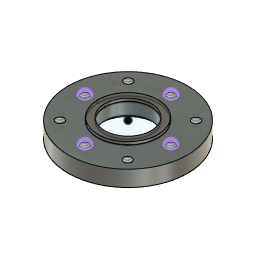
Driveshaft_adapter v1 (Autodesk Fusion 360 design; units mm, degrees)
Autodesk Fusion 360 part; units mm, degrees
note: some values were not read from the file. Set by a fixed rule: which sketch regions a step uses.
sketch "Big end" plane through (0, 0, 0) normal (0, 0, 1) x (1, 0, 0)
  circle A0 centre (0, 0) radius 75
  circle A1 centre (0, 0) radius 60.5 construction
  line L0 (-42.6, 42.9592) -> (42.6, 42.9592) construction
  line L1 (42.6, 42.9592) -> (42.6, -42.2408) construction
  line L2 (42.6, -42.2408) -> (-42.6, -42.2408) construction
  line L3 (-42.6, -42.2408) -> (-42.6, 42.9592) construction
  line L4 (42.6, 42.9592) -> (0, 0) construction
  line L5 (0, 0) -> (60.5, 0) construction
  circle A2 centre (-42.6, 42.9592) radius 6
  circle A3 centre (-42.9592, -42.6) radius 6
  circle A4 centre (42.6, -42.9592) radius 6
  circle A5 centre (42.9592, 42.6) radius 6
  circle A6 centre (0, 0) radius 54 construction
  circle A7 centre (54, 0) radius 6
  circle A8 centre (0, 54) radius 6
  circle A9 centre (-54, 0) radius 6
  circle A10 centre (0, -54) radius 6
  dimension "d1" = 150
  dimension "d2" = 121
  dimension "d4" = 85.2
  dimension "d5" = 85.2
  dimension "d6" = 12
  dimension "d8" = 360
  dimension "d15" = 108
  dimension "d16" = 12
  dimension "d18" = 360
  constraint coincident A0.centre A1.centre
  constraint concentric A0 A1
  constraint horizontal L0
  constraint vertical L1
  constraint horizontal L2
  constraint vertical L3
  constraint coincident A1 L0.start
  constraint coincident A1 L0.end
  constraint coincident A1 L5.end
  constraint perpendicular L1 L5
  constraint coincident L0.start L3.end
  constraint concentric A1 A6
  constraint coincident A6 A7.centre
  constraint coincident L5 A7.centre
  measures "d1" diameter of A0
  measures "d2" diameter of A1
  measures "d4" distance of L0.start L0.end
  measures "d5" distance of L0.start L2.end
  measures "d6" diameter of A2
  measures "d15" diameter of A6
  measures "d16" diameter of A7
extrude "Extrude1" add sketch "Big end" along normal blind 20 makes body 1
sketch "Big locating feature" plane through (0, 0, 20) normal (0, 0, 1) x (-1, 0, 0)
  circle A0 centre (42.6, -42.9592) radius 6
  circle A1 centre (-42.6, 42.9592) radius 6
  circle A2 centre (-42.9592, -42.6) radius 6
  circle A3 centre (42.9592, 42.6) radius 6
  circle A4 centre (0, 0) radius 75
  circle A5 centre (0, 0) radius 37.75
  circle A6 centre (0, -54) radius 6
  circle A7 centre (0, 54) radius 6
  circle A8 centre (54, 0) radius 6
  circle A9 centre (-54, 0) radius 6
  circle A10 centre (0, 0) radius 29.25
  dimension "d11" = 75.5
  dimension "d32" = 58.5
  constraint concentric A4 A5
  constraint concentric A5 A10
  measures "d11" diameter of A5
  measures "d32" diameter of A10
extrude "Extrude2" add sketch "Big locating feature" along normal blind 3.5 contours A5 | A10 bodies 1
sketch "Small end" plane through (0, 0, 0) normal (0, 0, -1) x (1, 0, 0)
  circle A0 centre (-42.6, -42.9592) radius 6
  circle A1 centre (42.6, 42.9592) radius 6
  circle A2 centre (42.9592, -42.6) radius 6
  circle A3 centre (-42.9592, 42.6) radius 6
  circle A4 centre (0, 0) radius 75
  circle A5 centre (0, -54) radius 6
  circle A6 centre (0, 54) radius 6
  circle A7 centre (-54, 0) radius 6
  circle A8 centre (54, 0) radius 6
  circle A9 centre (0, 0) radius 34.25
  dimension "d20" = 68.5
  constraint concentric A4 A9
  measures "d20" diameter of A9
extrude "Extrude3" cut sketch "Small end" against normal blind 5 contours A9 bodies 1
thread "Thread1" "ISO Metric profile 12.0 M12x1.75 6H" major diameter 12.2265 minor diameter 10.2735 pitch 1.75 angle 60 resizes the face on face at (-48.0075, -0.2991, 13.3333) on bodies 1
thread "Thread2" "ISO Metric profile 12.0 M12x1.75 6H" major diameter 12.2265 minor diameter 10.2735 pitch 1.75 angle 60 resizes the face on face at (-36.6075, 43.2582, 6.6667) on bodies 1
thread "Thread3" "ISO Metric profile 12.0 M12x1.75 6H" major diameter 12.2265 minor diameter 10.2735 pitch 1.75 angle 60 resizes the face on face at (5.9925, 54.2991, 6.6667) on bodies 1
thread "Thread4" "ISO Metric profile 12.0 M12x1.75 6H" major diameter 12.2265 minor diameter 10.2735 pitch 1.75 angle 60 resizes the face on face at (48.9517, 42.8991, 6.6667) on bodies 1
thread "Thread5" "ISO Metric profile 12.0 M12x1.75 6H" major diameter 12.2265 minor diameter 10.2735 pitch 1.75 angle 60 resizes the face on face at (59.9925, 0.2991, 6.6667) on bodies 1
thread "Thread6" "ISO Metric profile 12.0 M12x1.75 6H" major diameter 12.2265 minor diameter 10.2735 pitch 1.75 angle 60 resizes the face on face at (48.5925, -42.6601, 6.6667) on bodies 1
thread "Thread7" "ISO Metric profile 12.0 M12x1.75 6H" major diameter 12.2265 minor diameter 10.2735 pitch 1.75 angle 60 resizes the face on face at (5.9925, -53.7009, 6.6667) on bodies 1
thread "Thread8" "ISO Metric profile 12.0 M12x1.75 6H" major diameter 12.2265 minor diameter 10.2735 pitch 1.75 angle 60 resizes the face on face at (-36.9666, -42.3009, 6.6667) on bodies 1
sketch "waterjet outline" plane through (0, 0, 0) normal (0, 0, -1) x (1, 0, 0)
  circle A0 centre (0, 0) radius 34.25
  circle A1 centre (0, 0) radius 75
  circle A2 centre (0, 0) radius 76.2
  circle A3 centre (0, -54) radius 4.5
  circle A4 centre (54, 0) radius 4.5
  circle A5 centre (0, 54) radius 4.5
  circle A6 centre (-54, 0) radius 4.5
  circle A7 centre (-42.6, -42.9592) radius 4.5
  circle A8 centre (42.9592, -42.6) radius 4.5
  circle A9 centre (42.6, 42.9592) radius 4.5
  circle A10 centre (-42.9592, 42.6) radius 4.5
  circle A11 centre (-54, 0) radius 5.1368
  circle A12 centre (-42.6, -42.9592) radius 5.1368
  circle A13 centre (0, -54) radius 5.1368
  circle A14 centre (42.9592, -42.6) radius 5.1368
  circle A15 centre (42.6, 42.9592) radius 5.1368
  circle A16 centre (54, 0) radius 5.1368
  circle A17 centre (-42.9592, 42.6) radius 5.1368
  circle A18 centre (0, 54) radius 5.1368
  dimension "d23" = 152.4
  dimension "d24" = 9
  dimension "d26" = 360
  dimension "d27" = 9
  dimension "d29" = 360
  constraint concentric A0 A2
  constraint concentric A3 A13
  constraint concentric A7 A12
  measures "d23" diameter of A2
  measures "d24" diameter of A3
  measures "d27" diameter of A7
extrude "Extrude4" add sketch "waterjet outline" against normal blind 25.4 separate body contours A0 | A1 | A2 | A11 | A12 | A13 | A14 | A15 | A16 | A17 | A18 makes body 2
move_body "Move2" bodies 2 to x (1, 0, 0) y (0, 1, 0) z (0, 0, 1) at (0, 0, -0.95)
extrude "Extrude5" cut sketch "Big locating feature" along normal through all and the other way through all contours A10 bodies 1
hidden bodies 2
equation "d8 = 360.0 °"
equation "d18 = 360.0 °"
equation "d23 = 6\""
equation "d26 = 360.0 °"
equation "d29 = 360.0 °"
equation "d30 = -1\""
equation "d34 = 0.0 °"
named bodies: "driveshaft adapter", "waterjet stock"
